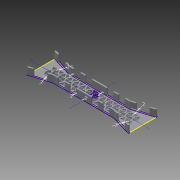
# Autodesk Inventor part: BandMiddle
Saved by Autodesk Inventor 2014 SP1 (Build 180222100, 222)
## iProperties
Created: 2015-03-16
Part Number: BandMiddle
Material: Generic
Document SubType Name: Modeling
Designer: Erin
Density: 1 g/cm^3
Appearance: Default
Author: Erin
Autodesk Inventor part; units mm, degrees
ref_plane "YZ Plane" through (0, 0, 0) normal (1, 0, 0) x (0, 1, 0)
ref_plane "XZ Plane" through (0, 0, 0) normal (0, 1, 0) x (-1, 0, 0)
ref_plane "XY Plane" through (0, 0, 0) normal (0, 0, 1) x (1, 0, 0)
sketch "Block1" plane through (0, 0, 0) normal (0, 0, 1) x (1, 0, 0)
  line L0 (-5.6547, 8.5) -> (0.3453, 8.5)
  line L1 (0.3453, 8.5) -> (-2.6547, 3.3038)
  line L2 (-2.6547, 3.3038) -> (-5.6547, 8.5)
  line L3 (-0.3453, 3.3038) -> (2.6547, 8.5)
  line L4 (5.6547, 3.3038) -> (-0.3453, 3.3038)
  line L5 (2.6547, 8.5) -> (5.6547, 3.3038)
  line L6 (-5.6547, 8.5) -> (5.6547, 8.5) construction
  line L7 (5.6547, 8.5) -> (5.6547, 3.3038) construction
  line L8 (5.6547, 3.3038) -> (-5.6547, 3.3038) construction
  line L9 (-5.6547, 3.3038) -> (-5.6547, 8.5) construction
  line L10 (0, 8.5) -> (0, 3.3038) construction
  line L11 (5.6547, 5.9019) -> (-5.6547, 5.9019) construction
  point P0 (0.0717, 5.9721)
  point P1 (-2.6547, 6.7679)
  point P2 (2.6547, 5.0359)
  dimension "d12" = 6
  dimension "d13" = 6
  dimension "d14" = 2
  measures "d12" distance of L0.start L0.end
  measures "d13" distance of L4.start L4.end
  measures "d14" distance between parallel lines of L1 L3
sketch "Sketch1" plane through (0, 0, 0) normal (0, 0, 1) x (1, 0, 0)
  line L0 (-75, 12.5) -> (75, 12.5)
  line L1 (75, 12.5) -> (75, -12.5)
  line L2 (75, -12.5) -> (-75, -12.5)
  line L3 (-75, -12.5) -> (-75, 12.5)
  line L4 (-80.4298, 21.5) -> (84.2578, 21.5) construction
  line L5 (84.2578, 21.5) -> (84.2578, -21.5) construction
  line L6 (84.2578, -21.5) -> (-80.4298, -21.5) construction
  line L7 (-80.4298, -21.5) -> (-80.4298, 21.5) construction
  line L8 (-75, 12.5) -> (-75, 21.5)
  line L9 (-75, -12.5) -> (-75, -21.5)
  line L10 (75, 12.5) -> (75, 21.5)
  line L11 (75, -12.5) -> (75, -21.5)
  line L12 (-45, 30.8502) -> (-45, -34.1581) construction
  line L13 (45, 32.7571) -> (45, -34.1581) construction
  line L14 (0, 40.2114) -> (0, -38.1453) construction
  line L15 (-75, 21.5) -> (-45, 12.5)
  line L16 (-75, -21.5) -> (-45, -12.5)
  line L17 (45, -12.5) -> (75, -21.5)
  line L18 (45, 12.5) -> (75, 21.5)
  line L19 (-75, 10) -> (-90, 10)
  line L20 (-90, 10) -> (-90, -10)
  line L21 (-90, -10) -> (-75, -10)
  line L22 (-75, -10) -> (-75, 10)
  line L23 (75, 10) -> (90, 10)
  line L24 (90, 10) -> (90, -10)
  line L25 (90, -10) -> (75, -10)
  line L26 (75, -10) -> (75, 10)
  point P0 (0, 0)
  point P1 (-75, 0)
  point P2 (0, 12.5)
  point P3 (-80.4298, 0)
  point P4 (-90, 0)
  point P5 (90, 0)
  dimension "d0" = 150
  dimension "d1" = 25
  dimension "d2" = 43
  dimension "d3" = 45
  dimension "d4" = 45
  dimension "d5" = 15
  dimension "d6" = 20
  dimension "d7" = 15
  dimension "d8" = 20
  constraints: 54 end point, 14 point on line, 11 parallel, 8 perpendicular, 5 midpoint, 4 horizontal, 4 horizontal alignment, 1 vertical, 1 vertical alignment
  measures "d0" distance of L1.end L2.end
  measures "d1" distance of L0.end L1.end
  measures "d2" distance of L6.end L4.start
  measures "d3" distance between parallel lines of L14 L12
  measures "d4" distance between parallel lines of L13 L14
  measures "d5" distance of L21.end L20.end
  measures "d6" distance of L20.end L19.end
  measures "d7" distance of L24.end L25.end
  measures "d8" distance of L23.end L24.end
extrude "Extrusion1" add sketch "Sketch1" along normal blind 0.6 contours L8 L15 L0 | L0 L1 L2 L3 | L18 L10 L0 | L2 L16 L9 | L2 L11 L17
sketch "Sketch2" plane through (0, 0, 0.6) normal (0, 0, 1) x (1, 0, 0)
  line L0 (75, -21.5) -> (75, 21.5) projected
  line L1 (45, 12.5) -> (-45, 12.5) projected
  line L2 (-75, 21.5) -> (-75, -21.5) projected
  line L3 (-45.2935, 10.5) -> (45.2935, 10.5)
  line L4 (45.2935, 10.5) -> (75, 19.4119)
  line L5 (75, -19.4119) -> (45.2935, -10.5)
  line L6 (45.2935, -10.5) -> (-45.2935, -10.5)
  line L7 (-45.2935, -10.5) -> (-75, -19.4119)
  line L8 (-75, 19.4119) -> (-45.2935, 10.5)
  line L9 (0, 35.8937) -> (0, -33.7191) construction
  line L10 (-93.0095, 0) -> (84.9368, 0) construction
  line L11 (-45, 12.5) -> (-75, 21.5) projected
  line L12 (-75, -21.5) -> (-45, -12.5) projected
  line L13 (-45, -12.5) -> (45, -12.5) projected
  line L14 (45, -12.5) -> (75, -21.5) projected
  line L15 (-75, -19.4119) -> (-75, -21.5)
  line L16 (-75, -21.5) -> (-45, -12.5)
  line L17 (-45, -12.5) -> (45, -12.5)
  line L18 (45, -12.5) -> (75, -21.5)
  line L19 (75, -21.5) -> (75, -19.4119)
  line L20 (75, 19.4119) -> (75, 21.5)
  line L21 (75, 21.5) -> (45, 12.5)
  line L22 (45, 12.5) -> (-45, 12.5)
  line L23 (-45, 12.5) -> (-75, 21.5)
  line L24 (-75, 21.5) -> (-75, 19.4119)
  line L25 (75, 21.5) -> (45, 12.5) projected
  line L26 (-5.6547, 8.5) -> (0.3453, 8.5)
  line L27 (0.3453, 8.5) -> (-2.6547, 3.3038)
  line L28 (-2.6547, 3.3038) -> (-5.6547, 8.5)
  line L29 (-0.3453, 3.3038) -> (2.6547, 8.5)
  line L30 (5.6547, 3.3038) -> (-0.3453, 3.3038)
  line L31 (2.6547, 8.5) -> (5.6547, 3.3038)
  line L32 (-5.6547, 8.5) -> (5.6547, 8.5) construction
  line L33 (5.6547, 8.5) -> (5.6547, 3.3038) construction
  line L34 (5.6547, 3.3038) -> (-5.6547, 3.3038) construction
  line L35 (-5.6547, 3.3038) -> (-5.6547, 8.5) construction
  line L36 (0, 8.5) -> (0, 3.3038) construction
  line L37 (5.6547, 5.9019) -> (-5.6547, 5.9019) construction
  line L38 (5.6547, 2.5981) -> (-0.3453, 2.5981)
  line L39 (-0.3453, 2.5981) -> (2.6547, -2.5981)
  line L40 (2.6547, -2.5981) -> (5.6547, 2.5981)
  line L41 (0.3453, -2.5981) -> (-2.6547, 2.5981)
  line L42 (-5.6547, -2.5981) -> (0.3453, -2.5981)
  line L43 (-2.6547, 2.5981) -> (-5.6547, -2.5981)
  line L44 (5.6547, 2.5981) -> (-5.6547, 2.5981) construction
  line L45 (-5.6547, 2.5981) -> (-5.6547, -2.5981) construction
  line L46 (-5.6547, -2.5981) -> (5.6547, -2.5981) construction
  line L47 (5.6547, -2.5981) -> (5.6547, 2.5981) construction
  line L48 (0, 2.5981) -> (0, -2.5981) construction
  line L49 (-5.6547, 0) -> (5.6547, 0) construction
  line L50 (-5.6547, -3.3038) -> (0.3453, -3.3038)
  line L51 (0.3453, -3.3038) -> (-2.6547, -8.5)
  line L52 (-2.6547, -8.5) -> (-5.6547, -3.3038)
  line L53 (-0.3453, -8.5) -> (2.6547, -3.3038)
  line L54 (5.6547, -8.5) -> (-0.3453, -8.5)
  line L55 (2.6547, -3.3038) -> (5.6547, -8.5)
  line L56 (-5.6547, -3.3038) -> (5.6547, -3.3038) construction
  line L57 (5.6547, -3.3038) -> (5.6547, -8.5) construction
  line L58 (5.6547, -8.5) -> (-5.6547, -8.5) construction
  line L59 (-5.6547, -8.5) -> (-5.6547, -3.3038) construction
  line L60 (0, -3.3038) -> (0, -8.5) construction
  line L61 (5.6547, -5.9019) -> (-5.6547, -5.9019) construction
  point P0 (0, 0)
  dimension "d11" = 2
  dimension "d15" = 2
  dimension "d16" = 2
  dimension "d36" = 2
  dimension "d37" = 2
  dimension "d38" = 2
  dimension "d39" = 2
  dimension "d40" = 2
  constraints: 36 end point, 6 collinear, 5 parallel, 5 vertical, 4 perpendicular, 4 point on line, 3 horizontal
  measures "d11" distance between parallel lines of L3 L1
  measures "d36" distance between parallel lines of L6 L13
  measures "d37" distance between parallel lines of L11 L8
  measures "d38" distance between parallel lines of L12 L7
  measures "d39" distance between parallel lines of L14 L5
  measures "d40" distance between parallel lines of L4 L25
extrude "Extrusion2" cut sketch "Sketch2" against normal blind 4 contours L26 L27 L28 | L29 L31 L30 | L40 L39 L38 | L42 L43 L41 | L50 L51 L52 | L53 L55 L54
pattern_linear "Rectangular Pattern1" count 7 spacing 10 along (-1, 0, 0) count 7 spacing 10 along (1, 0, 0) of "Extrusion2"
extrude "Extrusion3" add sketch "Sketch2" along normal blind 10 contours L14 L13 L12 L2 L7 L6 L5 L0 | L4 L3 L8 L2 L11 L1 L21 L0
sketch "Sketch3" plane through (0, 0, 0) normal (0, 1, 0) x (-1, 0, 0)
  line L0 (93.0095, 0.6) -> (-84.9368, 0.6) construction
  line L1 (-68, 15.7418) -> (-52, 15.7418)
  line L2 (-52, 15.7418) -> (-52, 0.6)
  line L3 (-52, 0.6) -> (-68, 0.6)
  line L4 (-68, 0.6) -> (-68, 15.7418)
  line L5 (-38, 0.6) -> (-28, 0.6)
  line L6 (-28, 0.6) -> (-28, 15.7418)
  line L7 (-28, 15.7418) -> (-38, 15.7418)
  line L8 (-38, 15.7418) -> (-38, 0.6)
  line L9 (-45, 0) -> (-45, 0.6) projected
  line L10 (45, 0) -> (45, 0.6) projected
  line L11 (-75, 0) -> (-75, 0.6) projected
  line L12 (75, 0) -> (75, 0.6) projected
  line L13 (-21, 0.6) -> (-11, 0.6)
  line L14 (-11, 0.6) -> (-11, 15.7418)
  line L15 (-11, 15.7418) -> (-21, 15.7418)
  line L16 (-21, 15.7418) -> (-21, 0.6)
  point P0 (0, 0)
  point P1 (-45, 10.6)
  point P2 (45, 10.6)
  point P3 (-75, 10.6)
  point P4 (75, 10.6)
  dimension "d28" = 10
  dimension "d29" = 7
  dimension "d30" = 7
  dimension "d31" = 10
  dimension "d32" = 7
  dimension "d35" = 7
  constraints: 24 end point, 6 parallel, 3 horizontal, 3 perpendicular, 4 other
  measures "d28" distance of L6.end L7.end
  measures "d29" distance between parallel lines of L11 L4
  measures "d30" distance between parallel lines of L9 L8
  measures "d31" distance of L14.end L15.end
  measures "d32" distance between parallel lines of L6 L16
  measures "d35" distance between parallel lines of L2 L9
extrude "Extrusion4" cut sketch "Sketch3" along normal mid plane 50
mirror "Mirror1" about plane through (0, 0, 0) normal (1, 0, 0) of "Extrusion4"
body "Solid1"
